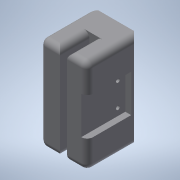
# Autodesk Inventor part: SP45V1 Plastico Roldana
Saved by Autodesk Inventor 2021.2 (Build 252289000, 289)
## iProperties
Created: 2026-09-01
Part Number: SP45V1 Plastico Roldana
Material: Generic
Document SubType Name: Modeling
Designer: nelso
Density: 1 g/cm^3
Appearance: Default
Author: nelso
Autodesk Inventor part; units mm, degrees
ref_plane "YZ Plane" through (0, 0, 0) normal (1, 0, 0) x (0, 1, 0)
ref_plane "XZ Plane" through (0, 0, 0) normal (0, 1, 0) x (-1, 0, 0)
ref_plane "XY Plane" through (0, 0, 0) normal (0, 0, 1) x (1, 0, 0)
sketch "Sketch1" plane through (0, 0, 0) normal (0, 1, 0) x (-1, 0, 0)
  line L0 (-20, 40) -> (20, 40)
  line L1 (20, 40) -> (20, -40)
  line L2 (20, -40) -> (-20, -40)
  line L3 (-20, -40) -> (-20, 40)
  line L4 (-20, 40) -> (20, -40) construction
  line L5 (20, 40) -> (-20, -40) construction
  point P0 (0, 0)
  dimension "d0" = 40
  dimension "d1" = 80
  constraints: 12 end point, 2 midpoint, 2 parallel, 1 horizontal, 1 perpendicular
  measures "d0" distance of L1.end L2.end
  measures "d1" distance of L0.end L1.end
extrude "Extrusion1" add sketch "Sketch1" along normal mid plane 45
sketch "Sketch2" plane through (0, -22.5, 0) normal (0, -1, 0) x (1, 0, 0)
  line L0 (20, -40) -> (-20, -40) projected
  line L1 (3, 40) -> (-3, 40)
  line L2 (-3, 40) -> (-3, -40)
  line L3 (-3, -40) -> (3, -40)
  line L4 (3, -40) -> (3, 40)
  line L5 (3, 40) -> (-3, -40) construction
  line L6 (-3, 40) -> (3, -40) construction
  point P0 (0, 0)
  dimension "d4" = 6
  constraints: 12 end point, 2 midpoint, 2 parallel, 1 horizontal, 1 perpendicular, 1 point on line
  measures "d4" distance of L3.end L2.end
extrude "Extrusion2" cut sketch "Sketch2" against normal blind 25
sketch "Sketch3" plane through (20, -22.5, -40) normal (1, 0, 0) x (0, 0, -1)
  line L0 (-40, 22.5) -> (-56, 22.5)
  line L1 (-80, 0) -> (0, 0) projected
  line L2 (-56, 22.5) -> (-24, 22.5)
  line L3 (-24, 22.5) -> (-24, 0)
  line L4 (-24, 0) -> (-56, 0)
  line L5 (-56, 0) -> (-56, 22.5)
  line L6 (-56, 22.5) -> (-24, 22.5)
  line L7 (-24, 22.5) -> (-24, 37.5)
  line L8 (-24, 37.5) -> (-56, 37.5)
  line L9 (-56, 37.5) -> (-56, 22.5)
  line L10 (-80, 25) -> (0, 25) projected
  line L11 (0, 25) -> (-80, 25) projected
  line L12 (-24, 25) -> (-24, 37.5)
  dimension "d7" = 16
  dimension "d8" = 32
  dimension "d9" = 15
  constraints: 20 end point, 4 parallel, 3 horizontal, 3 point on line, 2 perpendicular, 1 collinear
  measures "d7" distance of L0.start L0.end
  measures "d8" distance of L3.end L4.end
  measures "d9" distance of L7.end L6.end
extrude "Extrusion3" cut sketch "Sketch3" against normal blind 5
sketch "Sketch4" plane through (15, -22.5, -40) normal (1, 0, 0) x (0, 0, -1)
  line L0 (0, 25) -> (-80, 25) projected
  line L1 (-80, 25) -> (0, 25) projected
  line L2 (-40, 25) -> (-40, 31.25)
  line L3 (-56, 37.5) -> (-24, 37.5) projected
  line L4 (-40, 31.25) -> (-50, 31.25)
  point P0 (-40, 22.5)
  point P1 (-30, 31.25)
  dimension "d14" = 6.25
  dimension "d15" = 10
  constraints: 4 end point, 2 perpendicular, 1 coincident, 1 midpoint, 1 symmetric about line
  measures "d14" distance of L2.start L2.end
  measures "d15" distance of L2.end L4.end
hole "Hole1" at (15, 8.75, 10) at (15, 8.75, -10) direction (-1, 0, 0) diameter 3.2 depth 8 tip angle 118 clearance for "Countersunk Flat Head Screw ISO 2009/7046" size "M3" standard "ISO"
chamfer "Chamfer1" distance 5 angle 45 2 edges at (20, 22.5, 0) (-20, 22.5, 0)
chamfer "Chamfer2" distance 0.3 angle 45 2 edges at (0, 22.5, 40) (0, 22.5, -40)
fillet "Fillet1" radius 5 15 edges at (20, -2.5, 40) (-20, -2.5, 40) (20, -2.5, -40) (-20, -2.5, -40) (3, -10, -40) (-3, -10, -40) (-3, -10, 40) (3, -10, 40) (-20, -22.5, 0) (-11.5, -22.5, 40) (-11.5, -22.5, -40) (11.5, -22.5, -40) (20, -22.5, -28) (20, -22.5, 28) (11.5, -22.5, 40)
body "Solid1"
